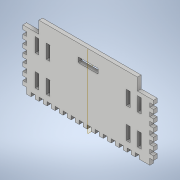
# Autodesk Inventor part: Side_one
Saved by Autodesk Inventor 2020 (Build 240168000, 168)
## iProperties
Created: 2019-12-17
Part Number: Side_one
Material: Generic
Document SubType Name: Modeling
Designer: fabfarm
Density: 1 g/cm^3
Appearance: Default
Author: fabfarm
Autodesk Inventor part; units mm, degrees
ref_plane "YZ Plane" through (0, 0, 0) normal (1, 0, 0) x (0, 1, 0)
ref_plane "XZ Plane" through (0, 0, 0) normal (0, 1, 0) x (-1, 0, 0)
ref_plane "XY Plane" through (0, 0, 0) normal (0, 0, 1) x (1, 0, 0)
sketch "Sketch1" plane through (0, 0, 0) normal (0, 0, 1) x (1, 0, 0)
  line L0 (0, 0) -> (-652, 0)
  line L1 (-652, 0) -> (-652, 350)
  line L2 (-652, 350) -> (0, 350)
  line L3 (0, 350) -> (0, 0)
  dimension "d0" = 350
  dimension "d1" = 652
  constraints: 8 end point, 2 parallel, 1 horizontal, 1 perpendicular
  measures "d0" distance of L2.end L0.start
  measures "d1" distance of L0.start L0.end
extrude "Extrusion1" add sketch "Sketch1" along normal blind 18.55
sketch "Sketch2" plane through (0, 0, 18.55) normal (0, 0, 1) x (1, 0, 0)
  line L0 (-652, 350) -> (-652, 0) projected
  line L1 (-652, 310) -> (-633.45, 310)
  line L2 (-633.45, 310) -> (-633.45, 290)
  line L3 (-633.45, 290) -> (-652, 290)
  line L4 (-652, 290) -> (-652, 310)
  line L5 (0, 350) -> (-652, 350) projected
  line L6 (-652, 270) -> (-633.45, 270)
  line L7 (-633.45, 270) -> (-633.45, 250)
  line L8 (-633.45, 250) -> (-652, 250)
  line L9 (-652, 250) -> (-652, 270)
  line L10 (-652, 230) -> (-633.45, 230)
  line L11 (-633.45, 230) -> (-633.45, 210)
  line L12 (-633.45, 210) -> (-652, 210)
  line L13 (-652, 210) -> (-652, 230)
  line L14 (-652, 190) -> (-633.45, 190)
  line L15 (-633.45, 190) -> (-633.45, 170)
  line L16 (-633.45, 170) -> (-652, 170)
  line L17 (-652, 170) -> (-652, 190)
  line L18 (-652, 150) -> (-633.45, 150)
  line L19 (-633.45, 150) -> (-633.45, 130)
  line L20 (-633.45, 130) -> (-652, 130)
  line L21 (-652, 130) -> (-652, 150)
  line L22 (-652, 110) -> (-633.45, 110)
  line L23 (-633.45, 110) -> (-633.45, 90)
  line L24 (-633.45, 90) -> (-652, 90)
  line L25 (-652, 90) -> (-652, 110)
  line L26 (-652, 70) -> (-633.45, 70)
  line L27 (-633.45, 70) -> (-633.45, 50)
  line L28 (-633.45, 50) -> (-652, 50)
  line L29 (-652, 50) -> (-652, 70)
  line L30 (-652, 350) -> (-633.45, 350)
  line L31 (-633.45, 350) -> (-633.45, 330)
  line L32 (-633.45, 330) -> (-652, 330)
  line L33 (-652, 330) -> (-652, 350)
  line L34 (-652, 30) -> (-633.45, 30)
  line L35 (-633.45, 30) -> (-633.45, 10)
  line L36 (-633.45, 10) -> (-652, 10)
  line L37 (-652, 10) -> (-652, 30)
  point P0 (0, 0)
  dimension "d4" = 40
  dimension "d5" = 20
  dimension "d6" = 18.55
  dimension "d9" = 40
  dimension "d16" = 20
  dimension "d17" = 18.55
  constraints: 72 end point, 4 parallel, 2 horizontal, 2 perpendicular, 1 point on line, 1 vertical, 56 other
  measures "d4" distance between parallel lines of L5 L1
  measures "d5" distance of L1.end L2.end
  measures "d6" distance of L1.start L1.end
  measures "d9" distance of L1.start L6.start
  measures "d16" distance between parallel lines of L32 L5
  measures "d17" distance between parallel lines of L33 L31
extrude "Extrusion2" cut sketch "Sketch2" against normal blind 18.55
ref_plane "Work Plane1" through (-326, 0, 0) normal (1, 0, 0) x (0, 0, -1)
mirror "Mirror1" about plane through (-326, 0, 0) normal (1, 0, 0) of "Extrusion2"
sketch "Sketch3" plane through (0, 0, 18.55) normal (0, 0, 1) x (1, 0, 0)
  line L0 (-18.55, 350) -> (-633.45, 350) projected
  line L1 (-652, 290) -> (-572, 290)
  line L2 (-572, 290) -> (-572, 350)
  line L3 (-572, 350) -> (-652, 350)
  line L4 (-652, 350) -> (-652, 290)
  line L5 (-652, 330) -> (-652, 350) construction
  line L6 (-652, 350) -> (-633.45, 350) construction
  point P0 (0, 0)
  dimension "d19" = 80
  dimension "d22" = 60
  constraints: 12 end point, 3 perpendicular, 1 parallel, 1 point on line, 1 vertical
  measures "d19" distance of L3.end L2.end
  measures "d22" distance of L3.end L1.start
extrude "Extrusion3" cut sketch "Sketch3" against normal blind 18.55
mirror "Mirror2" about plane through (-326, 0, 0) normal (1, 0, 0) of "Extrusion3"
sketch "Sketch4" plane through (0, 0, 18.55) normal (0, 0, 1) x (1, 0, 0)
  line L0 (-652, 0) -> (0, 0) projected
  line L1 (-611, 0) -> (-591, 0)
  line L2 (-591, 0) -> (-591, 18.55)
  line L3 (-591, 18.55) -> (-611, 18.55)
  line L4 (-611, 18.55) -> (-611, 0)
  line L5 (-652, 50) -> (-652, 0) projected
  line L6 (-571, 0) -> (-551, 0)
  line L7 (-551, 0) -> (-551, 18.55)
  line L8 (-551, 18.55) -> (-571, 18.55)
  line L9 (-571, 18.55) -> (-571, 0)
  line L10 (-531, 0) -> (-511, 0)
  line L11 (-511, 0) -> (-511, 18.55)
  line L12 (-511, 18.55) -> (-531, 18.55)
  line L13 (-531, 18.55) -> (-531, 0)
  line L14 (-491, 0) -> (-471, 0)
  line L15 (-471, 0) -> (-471, 18.55)
  line L16 (-471, 18.55) -> (-491, 18.55)
  line L17 (-491, 18.55) -> (-491, 0)
  line L18 (-451, 0) -> (-431, 0)
  line L19 (-431, 0) -> (-431, 18.55)
  line L20 (-431, 18.55) -> (-451, 18.55)
  line L21 (-451, 18.55) -> (-451, 0)
  line L22 (-411, 0) -> (-391, 0)
  line L23 (-391, 0) -> (-391, 18.55)
  line L24 (-391, 18.55) -> (-411, 18.55)
  line L25 (-411, 18.55) -> (-411, 0)
  line L26 (-371, 0) -> (-351, 0)
  line L27 (-351, 0) -> (-351, 18.55)
  line L28 (-351, 18.55) -> (-371, 18.55)
  line L29 (-371, 18.55) -> (-371, 0)
  line L30 (-331, 0) -> (-311, 0)
  line L31 (-311, 0) -> (-311, 18.55)
  line L32 (-311, 18.55) -> (-331, 18.55)
  line L33 (-331, 18.55) -> (-331, 0)
  line L34 (-291, 0) -> (-271, 0)
  line L35 (-271, 0) -> (-271, 18.55)
  line L36 (-271, 18.55) -> (-291, 18.55)
  line L37 (-291, 18.55) -> (-291, 0)
  line L38 (-251, 0) -> (-231, 0)
  line L39 (-231, 0) -> (-231, 18.55)
  line L40 (-231, 18.55) -> (-251, 18.55)
  line L41 (-251, 18.55) -> (-251, 0)
  line L42 (-211, 0) -> (-191, 0)
  line L43 (-191, 0) -> (-191, 18.55)
  line L44 (-191, 18.55) -> (-211, 18.55)
  line L45 (-211, 18.55) -> (-211, 0)
  line L46 (-171, 0) -> (-151, 0)
  line L47 (-151, 0) -> (-151, 18.55)
  line L48 (-151, 18.55) -> (-171, 18.55)
  line L49 (-171, 18.55) -> (-171, 0)
  line L50 (-131, 0) -> (-111, 0)
  line L51 (-111, 0) -> (-111, 18.55)
  line L52 (-111, 18.55) -> (-131, 18.55)
  line L53 (-131, 18.55) -> (-131, 0)
  line L54 (-91, 0) -> (-71, 0)
  line L55 (-71, 0) -> (-71, 18.55)
  line L56 (-71, 18.55) -> (-91, 18.55)
  line L57 (-91, 18.55) -> (-91, 0)
  line L58 (0, 0) -> (0, 50) projected
  line L59 (-51, 0) -> (-31, 0)
  line L60 (-31, 0) -> (-31, 18.55)
  line L61 (-31, 18.55) -> (-51, 18.55)
  line L62 (-51, 18.55) -> (-51, 0)
  dimension "d23" = 41
  dimension "d24" = 20
  dimension "d25" = 18.55
  dimension "d28" = 40
  dimension "d33" = 71
  constraints: 120 end point, 2 horizontal, 2 parallel, 1 perpendicular, 1 point on line, 112 other
  measures "d23" distance between parallel lines of L5 L4
  measures "d24" distance of L2.end L3.end
  measures "d25" distance of L1.end L2.end
  measures "d28" distance of L1.start L6.start
  measures "d33" distance between parallel lines of L55 L58
extrude "Extrusion4" cut sketch "Sketch4" against normal blind 20 contours L4 L3 L2 L0 | L9 L8 L7 L0 | L13 L12 L11 L0 | L17 L16 L15 L0 | L21 L20 L19 L0 | L25 L24 L23 L0 | L29 L28 L27 L0 | L33 L32 L31 L0 | L37 L36 L35 L0 | L41 L40 L39 L0 | L45 L44 L43 L0 | L49 L48 L47 L0 | L53 L52 L51 L0 | L57 L56 L55 L0
sketch "Sketch5" plane through (0, 0, 18.55) normal (0, 0, 1) x (1, 0, 0)
  line L0 (-652, 30) -> (-633.45, 30)
  line L1 (-633.45, 30) -> (-633.45, 0)
  line L2 (-633.45, 0) -> (-652, 0)
  line L3 (-652, 0) -> (-652, 30)
  line L4 (-18.55, 30) -> (0, 30) projected
  line L5 (-18.55, 30) -> (0, 30)
  line L6 (0, 30) -> (0, 0)
  line L7 (0, 0) -> (-18.55, 0)
  line L8 (-18.55, 0) -> (-18.55, 30)
  line L9 (-633.45, 30) -> (-633.45, 10) projected
  line L10 (-652, 0) -> (-611, 0) projected
  constraints: 16 end point, 4 parallel, 2 collinear, 2 horizontal, 2 perpendicular
extrude "Extrusion5" cut sketch "Sketch5" against normal blind 20
sketch "Sketch6" plane through (0, 0, 18.55) normal (0, 0, 1) x (1, 0, 0)
  line L0 (-276, 265) -> (-376, 265)
  line L1 (-376, 265) -> (-376, 290)
  line L2 (-376, 290) -> (-276, 290)
  line L3 (-276, 290) -> (-276, 265)
  line L4 (-276, 265) -> (-376, 290) construction
  line L5 (-376, 265) -> (-276, 290) construction
  line L6 (-326, 420) -> (-326, -70) projected
  line L7 (-80, 350) -> (-572, 350) projected
  point P0 (0, 0)
  point P1 (-326, 277.5)
  dimension "d38" = 25
  dimension "d39" = 100
  dimension "d40" = 60
  constraints: 12 end point, 2 midpoint, 2 parallel, 1 horizontal, 1 perpendicular, 1 point on line
  measures "d38" distance of L0.end L1.end
  measures "d39" distance of L1.end L2.end
  measures "d40" distance between parallel lines of L7 L2
extrude "Extrusion6" cut sketch "Sketch6" against normal blind 20
fillet "Fillet1" radius 4 4 edges at (-276, 290, 9.275) (-276, 265, 9.275) (-376, 290, 9.275) (-376, 265, 9.275)
sketch "Sketch7" plane through (0, 0, 18.55) normal (0, 0, 1) x (1, 0, 0)
  line L0 (-590.55, 48.55) -> (-572, 48.55)
  line L1 (-572, 48.55) -> (-572, 118.55)
  line L2 (-572, 118.55) -> (-590.55, 118.55)
  line L3 (-590.55, 118.55) -> (-590.55, 48.55)
  line L4 (-534.9, 48.55) -> (-516.35, 48.55)
  line L5 (-516.35, 48.55) -> (-516.35, 118.55)
  line L6 (-516.35, 118.55) -> (-534.9, 118.55)
  line L7 (-534.9, 118.55) -> (-534.9, 48.55)
  line L8 (-611, 18.55) -> (-591, 18.55) projected
  line L9 (-633.45, 70) -> (-633.45, 50) projected
  line L10 (-572, 350) -> (-572, 290) projected
  point P0 (0, 0)
  dimension "d44" = 37.1
  dimension "d45" = 18.55
  dimension "d46" = 70
  dimension "d47" = 30
  constraints: 16 end point, 4 parallel, 2 collinear, 2 horizontal, 2 perpendicular, 2 point on line
  measures "d44" distance between parallel lines of L7 L1
  measures "d45" distance of L1.end L2.end
  measures "d46" distance of L2.end L0.start
  measures "d47" distance between parallel lines of L8 L0
extrude "Extrusion7" cut sketch "Sketch7" against normal blind 20
mirror "Mirror3" about plane through (-326, 0, 0) normal (1, 0, 0) of "Extrusion7"
sketch "Esquisse8" plane through (0, 0, 0) normal (0, 0, -1) x (-1, 0, 0)
  line L0 (80, 200) -> (61.45, 200)
  line L1 (61.45, 200) -> (61.45, 270)
  line L2 (61.45, 270) -> (80, 270)
  line L3 (80, 270) -> (80, 200)
  line L4 (117.1, 270) -> (135.65, 270)
  line L5 (135.65, 270) -> (135.65, 200)
  line L6 (135.65, 200) -> (117.1, 200)
  line L7 (117.1, 200) -> (117.1, 270)
  line L8 (61.45, 48.55) -> (61.45, 118.55) projected
  line L9 (80, 118.55) -> (80, 48.55) projected
  line L10 (117.1, 48.55) -> (117.1, 118.55) projected
  line L11 (135.65, 118.55) -> (135.65, 48.55) projected
  line L12 (0, 270) -> (18.55, 270) projected
  point P0 (0, 0)
  dimension "d51" = 70
  constraints: 16 end point, 5 collinear, 4 parallel, 2 horizontal, 2 perpendicular, 2 point on line
  measures "d51" distance of L0.end L1.end
extrude "Extrusion8" cut sketch "Esquisse8" against normal blind 20
mirror "Symétrie4" about plane through (-326, 0, 0) normal (1, 0, 0) of "Extrusion8"
body "Solid1"
